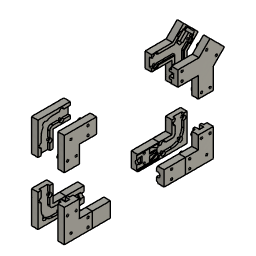
Gabellichtschranke Vorlage v11 (Autodesk Fusion 360 design; units mm, degrees)
Autodesk Fusion 360 part; units mm, degrees
note: some values were not read from the file. Chosen so that the rebuilt part matches the saved one: which bodies a step acts on; which face or edge a step refers to; which pieces of a blend or face edit are solid. Set by a fixed rule: which sketch regions a step uses.
(part 1 of 2)
sketch "Skizze1" plane through (0, 0, 0) normal (1, 0, 0) x (0, 1, 0)
  line L0 (0, 0) -> (80, 0)
  line L1 (80, 0) -> (80, -12)
  line L2 (80, -12) -> (0, -12)
  line L3 (0, -12) -> (0, 0)
  line L4 (0, -12) -> (80, -12)
  line L5 (80, -12) -> (80, -8)
  line L6 (80, -8) -> (0, -8)
  line L7 (0, -8) -> (0, -12)
  line L8 (0, 0) -> (80, 0)
  line L9 (80, 0) -> (80, -4)
  line L10 (0, -4) -> (0, 0)
  line L11 (0, -4) -> (80, -4)
  dimension "d1" = 80
  dimension "d2" = 12
  dimension "d3" = 4
  dimension "d4" = 4
  constraint horizontal L0
  constraint vertical L1
  constraint horizontal L2
  constraint vertical L3
  constraint coincident L0.start L3.end
  constraint horizontal L4
  constraint vertical L5
  constraint horizontal L6
  constraint vertical L7
  constraint coincident L1 L5.end
  constraint horizontal L8
  constraint vertical L9
  constraint vertical L10
  constraint coincident L1 L9.end
  constraint perpendicular L9 L11
  measures "d1" distance of L0.start L0.end
  measures "d2" distance of L0.start L2.end
  measures "d3" distance of L2.end L6.end
  measures "d4" distance of L0.start L10.start
extrude "Extrusion2" add sketch "Skizze1" along normal blind 6 makes body 1
sketch "Skizze2" plane through (0, 0, 0) normal (0, -1, 0) x (1, 0, 0)
  line L0 (0, 0) -> (0, -12)
  line L1 (0, -12) -> (6, -12)
  line L2 (6, -12) -> (6, 0)
  line L3 (6, 0) -> (0, 0)
  circle A0 centre (0, -6) radius 2
  circle A1 centre (0, -6) radius 2.5
  circle A2 centre (0, -6) radius 3
  dimension "d16" = 4
  dimension "d17" = 5
  dimension "d18" = 6
  constraint midpoint L0 A0.centre
  constraint concentric A0 A1
  constraint concentric A0 A2
  measures "d16" diameter of A0
  measures "d17" diameter of A1
  measures "d18" diameter of A2
extrude "Extrusion3" cut sketch "Skizze2" against normal blind 3 contours L0 A0 picked at (0.5038, -5.5634) bodies 1
extrude "Extrusion4" cut sketch "Skizze2" against normal blind 6 from surface at -3 contours L0 A1 A2 | L0 A0 A1 | L0 A0 picked at (0.9319, -8.6687) picked at (0.1186, -3.6751) picked at (0.5038, -5.5634) bodies 1
extrude "Extrusion5" cut sketch "Skizze2" against normal blind 0.8 from surface at -9 contours L0 A0 A1 | L0 A0 picked at (0.1186, -3.6751) picked at (0.5038, -5.5634) bodies 1
extrude "Extrusion6" cut sketch "Skizze2" against normal blind 7 from surface at -9.8 contours L0 A1 A2 | L0 A0 A1 | L0 A0 picked at (0.9319, -8.6687) picked at (0.1186, -3.6751) picked at (0.5038, -5.5634) bodies 1
sketch "Skizze3" plane through (0, 0, 0) normal (-1, 0, 0) x (0, -1, 0)
  line L0 (-9.8, -8.5) -> (-9.8, -9)
  line L1 (-9.8, -9) -> (-16.8, -9)
  line L2 (-16.8, -9) -> (-16.8, -3)
  line L3 (-16.8, -3) -> (-9.8, -3)
  line L4 (-9.8, -3) -> (-9.8, -3.5)
  line L5 (-9.8, -3.5) -> (-9, -3.5)
  line L6 (-9, -3.5) -> (-9, -3)
  line L7 (-9, -3) -> (-3, -3)
  line L8 (-3, -3) -> (-3, -4)
  line L9 (-3, -4) -> (0, -4)
  line L10 (0, -4) -> (0, 0)
  line L11 (0, 0) -> (-80, 0)
  line L12 (-80, 0) -> (-80, -12)
  line L13 (-80, -12) -> (0, -12)
  line L14 (0, -12) -> (0, -8)
  line L15 (0, -8) -> (-3, -8)
  line L16 (-3, -8) -> (-3, -9)
  line L17 (-3, -9) -> (-9, -9)
  line L18 (-9, -9) -> (-9, -8.5)
  line L19 (-9, -8.5) -> (-9.8, -8.5)
  line L20 (-16.8, -6) -> (-19.8, -6)
  line L21 (-19.8, -6) -> (-19.8, -8)
  line L22 (-19.8, -6) -> (-19.8, -4)
  line L23 (-19.8, -4) -> (-80, -4)
  line L24 (-19.8, -8) -> (-80, -8)
  line L25 (-19.8, -4) -> (-19.8, -2)
  line L26 (-19.8, -8) -> (-19.8, -10)
  line L27 (-19.8, -2) -> (-80, -2)
  line L28 (-19.8, -10) -> (-80, -10)
  line L29 (-19.8, -2) -> (-22.8, -2)
  circle A0 centre (-22.8, -2) radius 2
  line L30 (-22.8, -2) -> (-52.8, -2)
  circle A1 centre (-52.8, -2) radius 2
  line L31 (-19.8, -10) -> (-22.8, -10)
  line L32 (-22.8, -10) -> (-52.8, -10)
  circle A2 centre (-52.8, -10) radius 2
  circle A3 centre (-22.8, -10) radius 2
  circle A4 centre (-52.8, -2) radius 1
  circle A5 centre (-22.8, -2) radius 1
  circle A6 centre (-52.8, -10) radius 1
  circle A7 centre (-22.8, -10) radius 1
  circle A8 centre (-22.8, -2) radius 2.75
  circle A9 centre (-52.8, -2) radius 2.75
  circle A10 centre (-52.8, -10) radius 2.75
  circle A11 centre (-22.8, -10) radius 2.75
  dimension "d30" = 3
  dimension "d31" = 2
  dimension "d32" = 2
  dimension "d33" = 2
  dimension "d34" = 2
  dimension "d41" = 3
  dimension "d42" = 4
  dimension "d43" = 30
  dimension "d44" = 4
  dimension "d45" = 3
  dimension "d46" = 30
  dimension "d47" = 4
  dimension "d48" = 4
  dimension "d49" = 2
  dimension "d50" = 2
  dimension "d51" = 2
  dimension "d52" = 2
  dimension "d62" = 5.5
  dimension "d63" = 5.5
  dimension "d64" = 5.5
  dimension "d65" = 5.5
  constraint midpoint L2 L20.start
  constraint perpendicular L2 L20
  constraint perpendicular L1 L21
  constraint perpendicular L20 L22
  constraint coincident L12 L23.end
  constraint perpendicular L12 L23
  constraint coincident L12 L24.end
  constraint perpendicular L12 L24
  constraint perpendicular L23 L25
  constraint perpendicular L24 L26
  constraint coincident L12 L27.end
  constraint perpendicular L12 L27
  constraint coincident L12 L28.end
  constraint perpendicular L12 L28
  constraint perpendicular L25 L29
  constraint coincident L29.end A0.centre
  constraint parallel L27 L30
  constraint coincident L30.end A1.centre
  constraint perpendicular L26 L31
  constraint parallel L28 L32
  constraint coincident L32.end A2.centre
  constraint coincident L31.end L32.start
  constraint concentric A1 A4
  constraint concentric A0 A5
  constraint concentric A2 A6
  constraint concentric A3 A7
  constraint concentric A0 A8
  constraint concentric A4 A9
  constraint concentric A6 A10
  constraint concentric A3 A11
  measures "d30" distance of L20.start L20.end
  measures "d31" distance of L20.end L21.end
  measures "d32" distance of L20.end L22.end
  measures "d33" distance of L22.end L25.end
  measures "d34" distance of L21.end L26.end
  measures "d41" distance of L25.end L29.end
  measures "d42" diameter of A0
  measures "d43" distance of L29.end L30.end
  measures "d44" diameter of A1
  measures "d45" distance of L26.end L31.end
  measures "d46" distance of L31.end L32.end
  measures "d47" diameter of A2
  measures "d48" diameter of A3
  measures "d49" diameter of A4
  measures "d50" diameter of A5
  measures "d51" diameter of A6
  measures "d52" diameter of A7
  measures "d62" diameter of A8
  measures "d63" diameter of A9
  measures "d64" diameter of A10
  measures "d65" diameter of A11
extrude "Extrusion7" add sketch "Skizze3" along normal blind 2 contours L24 L26 L28 L31 A11 | L23 L25 L27 L29 A8 | L24 L28 L31 A3 A11 | L23 L27 L29 A0 A8 | L24 L28 L32 A3 A11 | L28 L31 L32 A3 A7 | L24 L28 L32 A10 A11 | L23 L27 A0 L30 A8 | L27 L29 A0 L30 A5 | L23 L27 L30 A8 A9 | L24 L28 L32 A2 A10 | L23 L27 L30 A1 A9 | L28 L31 L32 A7 | L24 L28 A2 A10 | L28 L32 A2 A6 | L12 L24 L28 A10 | L27 L29 L30 A5 | L23 L27 A1 A9 | L27 L30 A1 A4 | L12 L23 L27 A9 | L28 L32 A6 | L27 L30 A4 picked at (-22.9198, -8.3411) picked at (-22.9198, -3.6589) picked at (-23.3198, -9.5855) picked at (-52.9198, -8.3411) picked at (-22.1371, -2.0497) picked at (-52.9198, -3.6589) picked at (-52.3478, -9.5127) picked at (-52.1371, -2.0497) bodies 1
extrude "Extrusion8" cut sketch "Skizze3" against normal blind 2 contours L12 L21 L22 L23 L24 A8 A9 A10 A11 | L24 A11 | L23 A8 | L24 A10 | L23 A9 bodies 1
extrude "Extrusion9" cut 1 faces at (0.6667, 19.8, -6.6667) along direction (0, -1, 0) blind 6 on bodies 1 bodies 1
extrude "Extrusion10" add sketch "Skizze3" along normal blind 2 contours L28 L31 L32 A3 A7 | L27 L29 A0 L30 A5 | L28 L31 L32 A7 | L27 L29 L30 A5 | L28 L32 A2 A6 | L27 L30 A1 A4 | L28 L32 A6 | L27 L30 A4 picked at (-22.9198, -11.6589) picked at (-22.9198, -0.3411) picked at (-23.4629, -10.0497) picked at (-23.4629, -1.9503) picked at (-52.9198, -11.6589) picked at (-52.9198, -0.3411) picked at (-53.4629, -10.0497) picked at (-53.4629, -1.9503) bodies 1
extrude "Extrusion11" cut 1 faces at (4.6667, 80, -5.3333) along direction (0, -1, 0) blind 22 on bodies 1 bodies 1
copy_body "Körper kopieren/einfügen1" bodies 1 makes body 2
move_body "Verschieben1" bodies 2 to x (1, 0, 0) y (0, 1, 0) z (0, 0, 1) at (-33, 0, 0)
extrude "Extrusion12" cut 2 faces at (-35, 34.2, -8.6667) (-35, 42.8667, -3.3333) along direction (1, 0, 0) blind 4 on bodies 2 bodies 2
extrude "Extrusion13" cut sketch "Skizze3" along normal blind 100 from surface at -10 contours L28 L31 L32 A7 | L28 L31 L32 A7 | L27 L29 L30 A5 | L27 L29 L30 A5 | L28 L32 A6 | L28 L32 A6 | L27 L30 A4 | L27 L30 A4 bodies 1 2
extrude "Extrusion14" add 2 faces at (4, 26.9333, 0) (-30.3333, 7.6, 0) along direction (0, 0, 1) blind 1 on bodies 1 2 bodies 1 2
extrude "Extrusion15" add 2 faces at (4, 26.9333, -12) (-30.3333, 7.6, -12) along direction (0, 0, -1) blind 1 on bodies 1 2 bodies 1 2
extrude "Extrusion16" cut sketch "Skizze3" against normal blind 3 from surface at -3 contours L24 L28 L31 A3 A11 | L24 A11 | L23 A8 | L23 L27 L29 A0 A8 | L24 L28 L32 A3 A11 | L28 L31 L32 A3 A7 | L13 L28 L31 A3 A11 | L23 L27 A0 L30 A8 | L27 L29 A0 L30 A5 | L11 L27 L29 A0 A8 | L13 A11 | L28 L31 L32 A3 A7 | L13 L28 L32 A3 A11 | L24 L28 L32 A2 A10 | L24 A10 | L27 L29 A0 L30 A5 | L11 L27 A0 L30 A8 | L23 A9 | L23 L27 L30 A1 A9 | L11 A8 | L28 L31 L32 A7 | L28 L31 L32 A7 | L24 L28 A2 A10 | L28 L32 A2 A6 | L13 L28 L32 A2 A10 | L27 L29 L30 A5 | L27 L29 L30 A5 | L23 L27 A1 A9 | L27 L30 A1 A4 | L11 L27 L30 A1 A9 | L13 A10 | L28 L32 A2 A6 | L13 L28 A2 A10 | L27 L30 A1 A4 | L11 L27 A1 A9 | L11 A9 | L28 L32 A6 | L28 L32 A6 | L27 L30 A4 | L27 L30 A4 bodies 1
move_body "Verschieben2" bodies 2 to x (-1, 0, 0) y (0, 1, 0) z (0, 0, -1) at (-66, 0, -26)
move_body "Verschieben3" bodies 2 to x (1, 0, 0) y (0, 1, 0) z (0, 0, 1) at (33, 0, 14)
move_body "Verschieben4" bodies 2 to x (1, 0, 0) y (0, 1, 0) z (0, 0, 1) at (-12, 0, 0)
copy_body "Körper kopieren/einfügen2" bodies 1 makes body 3
move_body "Verschieben5" bodies 3 to x (1, 0, 0) y (0, 1, 0) z (0, 0, 1) at (-52, 0, 0)
extrude "Extrusion17" cut 1 faces at (-47.3352, 0, -6.0498) along direction (0, 1, 0) blind 18 on bodies 3 bodies 3
extrude "Extrusion18" add 1 faces at (-47.3333, 18, -5.3333) along direction (0, -1, 0) blind 18 on bodies 3 bodies 3
sketch "Skizze4" plane through (-52, 0, 0) normal (-1, 0, 0) x (0, -1, 0)
  line L0 (0, -8) -> (-19.8, -8)
  line L1 (-19.8, -8) -> (-19.8, -10)
  line L2 (-19.8, -10) -> (-20.8, -10)
  arc A0 (-24.8, -10) -> (-20.8, -10) centre (-22.8, -10) ccw
  line L3 (-24.8, -10) -> (-50.8, -10)
  arc A1 (-54.8, -10) -> (-50.8, -10) centre (-52.8, -10) ccw
  line L4 (-54.8, -10) -> (-58, -10)
  line L5 (-58, -10) -> (-58, -13)
  line L6 (-58, -13) -> (0, -13)
  line L7 (0, -13) -> (0, -8)
  line L8 (-16, -8) -> (-19.8, -8)
  line L9 (-19.8, -8) -> (-19.8, -4)
  line L10 (-19.8, -4) -> (-16, -4)
  line L11 (0, -4) -> (0, -8)
  line L12 (0, -6) -> (-19.8, -6) construction
  line L13 (0, -6) -> (-2, -6)
  line L14 (-2, -6) -> (-2, -8.75)
  line L15 (-2, -6) -> (-2, -3.25)
  line L16 (-2, -3.25) -> (-5, -3.25)
  line L17 (-5, -3.25) -> (-5, -8.75)
  line L18 (-5, -8.75) -> (-2, -8.75)
  line L19 (-2, -8.75) -> (-2, -3.25)
  line L20 (-5, -6) -> (-5, -7.25)
  line L21 (-5, -7.25) -> (-10, -7.25)
  line L22 (-10, -7.25) -> (-10, -4.75)
  line L23 (-10, -4.75) -> (-5, -4.75)
  line L24 (-5, -4.75) -> (-5, -7.25)
  line L25 (-5, -7.25) -> (-5, -8.25)
  line L26 (-5, -4.75) -> (-5, -3.75)
  line L27 (-5, -8.25) -> (-8, -8.25)
  line L28 (-5, -3.75) -> (-8, -3.75)
  line L29 (-9, -9.25) -> (-9, -10.25)
  line L30 (-10, -7.25) -> (-10, -9.25)
  line L31 (-11, -10.25) -> (-13, -10.25)
  line L32 (-14, -9.25) -> (-14, -7.25)
  line L33 (-10, -4.75) -> (-10, -2.75)
  line L34 (-9, -2.75) -> (-9, -1.75)
  line L35 (-11, -1.75) -> (-13, -1.75)
  line L36 (-14, -2.75) -> (-14, -7.25)
  line L37 (-10, -0.75) -> (-14, -0.75)
  line L38 (-15, -1.75) -> (-15, -3)
  line L39 (-10, -11.25) -> (-14, -11.25)
  line L40 (-15, -10.25) -> (-15, -9)
  line L41 (-14, -6) -> (-14, -6.75)
  line L42 (-14, -6) -> (-14, -5.25)
  line L43 (-16.8, -4) -> (-16.8, -8)
  line L44 (-14, -6.75) -> (-16.8, -6.75)
  line L45 (-14, -5.25) -> (-16.8, -5.25)
  arc A2 (-8, -8.25) -> (-9, -9.25) centre (-8, -9.25) ccw
  arc A3 (-11, -10.25) -> (-10, -9.25) centre (-11, -9.25) ccw
  arc A4 (-14, -9.25) -> (-13, -10.25) centre (-13, -9.25) ccw
  arc A5 (-15, -9) -> (-16, -8) centre (-16, -9) ccw
  arc A6 (-9, -2.75) -> (-8, -3.75) centre (-8, -2.75) ccw
  arc A7 (-10, -2.75) -> (-11, -1.75) centre (-11, -2.75) ccw
  arc A8 (-13, -1.75) -> (-14, -2.75) centre (-13, -2.75) ccw
  arc A9 (-16, -4) -> (-15, -3) centre (-16, -3) ccw
  arc A10 (-9, -1.75) -> (-10, -0.75) centre (-10, -1.75) ccw
  arc A11 (-14, -0.75) -> (-15, -1.75) centre (-14, -1.75) ccw
  arc A12 (-15, -10.25) -> (-14, -11.25) centre (-14, -10.25) ccw
  arc A13 (-10, -11.25) -> (-9, -10.25) centre (-10, -10.25) ccw
  point P0 (-19.8, -4)
  point P1 (-9, -8.25)
  point P2 (-9, -3.75)
  point P3 (-9, -11.25)
  point P4 (-10, -10.25)
  point P5 (-14, -10.25)
  point P6 (-10, -1.75)
  point P7 (-9, -0.75)
  point P8 (-14, -1.75)
  point P9 (-15, -0.75)
  dimension "d79" = 2
  dimension "d80" = 2.75
  dimension "d81" = 2.75
  dimension "d82" = 3
  dimension "d83" = 5.5
  dimension "d84" = 1.25
  dimension "d85" = 5
  dimension "d86" = 2.5
  dimension "d87" = 1
  dimension "d88" = 1
  dimension "d89" = 4
  dimension "d90" = 4
  dimension "d92" = 3
  dimension "d93" = 4
  dimension "d94" = 3
  dimension "d95" = 3
  dimension "d96" = 4
  dimension "d97" = 6
  dimension "d107" = 0.75
  dimension "d108" = 0.75
  dimension "d113" = 1
  dimension "d118" = 1
  constraint horizontal L8
  constraint vertical L9
  constraint horizontal L10
  constraint vertical L11
  constraint coincident P0 L9.end
  constraint coincident L0.start L7.end
  constraint midpoint L11 L12.start
  constraint midpoint L9 L12.end
  constraint perpendicular L11 L13
  constraint perpendicular L13 L14
  constraint perpendicular L12 L15
  constraint horizontal L16
  constraint vertical L17
  constraint horizontal L18
  constraint vertical L19
  constraint midpoint L17 L20.start
  constraint perpendicular L12 L20
  constraint horizontal L21
  constraint vertical L22
  constraint horizontal L23
  constraint vertical L24
  constraint perpendicular L21 L25
  constraint perpendicular L10 L26
  constraint perpendicular L25 L27
  constraint perpendicular L17 L28
  constraint perpendicular L8 L29
  constraint perpendicular L8 L30
  constraint perpendicular L30 L31
  constraint perpendicular L21 L32
  constraint perpendicular L10 L33
  constraint perpendicular L28 L34
  constraint perpendicular L33 L35
  constraint perpendicular L34 L37
  constraint vertical L38
  constraint perpendicular L29 L39
  constraint coincident L36 L41.start
  constraint coincident L12 L41.start
  constraint perpendicular L12 L41
  constraint perpendicular L12 L42
  constraint coincident L43 L44.end
  constraint perpendicular L36 L44
  constraint horizontal L45
  constraint coincident L43 L45.end
  constraint coincident P1 L29
  constraint coincident P1 L27
  constraint tangent L29 A2
  constraint tangent L27 A2
  constraint coincident P4 L31
  constraint coincident P4 L30
  constraint tangent L31 A3
  constraint tangent L30 A3
  constraint equal A2 A3
  constraint coincident P5 L31
  constraint coincident P5 L32
  constraint tangent L31 A4
  constraint tangent L32 A4
  constraint equal A2 A4
  constraint coincident L0.start L8
  constraint tangent L40 A5
  constraint tangent L8 A5
  constraint equal A2 A5
  constraint coincident P2 L28
  constraint coincident P2 L34
  constraint tangent L28 A6
  constraint tangent L34 A6
  constraint equal A2 A6
  constraint coincident P6 L33
  constraint coincident P6 L35
  constraint tangent L33 A7
  constraint tangent L35 A7
  constraint equal A2 A7
  constraint coincident P8 L35
  constraint coincident P8 L36
  constraint tangent L35 A8
  constraint tangent L36 A8
  constraint equal A2 A8
  constraint coincident L11.start L10
  constraint tangent L10 A9
  constraint tangent L38 A9
  constraint equal A2 A9
  constraint coincident P7 L34
  constraint coincident P7 L37
  constraint tangent L34 A10
  constraint tangent L37 A10
  constraint coincident P9 L37
  constraint coincident P9 L38
  constraint tangent L37 A11
  constraint tangent L38 A11
  constraint equal A10 A11
  constraint tangent L40 A12
  constraint tangent L39 A12
  constraint equal A10 A12
  constraint coincident P3 L39
  constraint coincident P3 L29
  constraint tangent L39 A13
  constraint tangent L29 A13
  constraint equal A10 A13
  measures "d79" distance of L12.start L13.end
  measures "d80" distance of L13.end L14.end
  measures "d81" distance of L13.end L15.end
  measures "d82" distance of L15.end L16.end
  measures "d83" distance of L15.end L14.end
  measures "d84" distance of L20.start L20.end
  measures "d85" distance of L20.end L21.end
  measures "d86" distance of L20.end L23.end
  measures "d87" distance of L20.end L25.end
  measures "d88" distance of L23.end L26.end
  measures "d89" distance of L25.end P1
  measures "d90" distance of L26.end P2
  measures "d92" distance of L21.end P4
  measures "d93" distance of P4 P5
  measures "d94" distance of L22.end P6
  measures "d95" distance of P2 P7
  measures "d96" distance of P6 P8
  measures "d97" distance of P7 P9
  measures "d107" distance of L41.start L41.end
  measures "d108" distance of L41.start L42.end
  measures "d113" radius of A2
  measures "d118" radius of A10
extrude "Extrusion19" add sketch "Skizze4" against normal blind 2 contours L0 L8 L9 L10 L43 bodies 3
extrude "Extrusion21" cut sketch "Skizze4" against normal blind 1 contours L0 L17 L25 L27 L29 L30 L31 L32 L39 L40 A2 A3 A4 A5 A12 A13 | L0 L17 L21 L25 L30 | L10 L17 L23 L26 L28 L33 L34 L35 L36 L37 L38 L43 L45 A6 A7 A8 A9 A10 A11 bodies 3
extrude "Extrusion22" cut sketch "Skizze4" against normal blind 2.5 contours L0 L14 L15 L16 L17 L19 L20 L24 L25 L26 | L0 L14 L17 L18 L19 L25 bodies 3
extrude "Extrusion23" cut sketch "Skizze4" against normal blind 2 contours L0 L8 L9 L10 L43 bodies 3
extrude "Extrusion25" add sketch "Skizze4" against normal blind 2 contours L36 L41 L42 L43 L44 L45 bodies 3
extrude "Extrusion26" add sketch "Skizze4" against normal blind 2 contours L0 L22 L30 L32 L33 L35 L36 L41 L42 A7 A8 | L17 L20 L21 L22 L23 L24 bodies 3
extrude "Extrusion27" add 2 faces at (-50, 8.3333, -7.5) (-50, 8.3333, -4.25) along direction (-1, 0, 0) blind 1 on bodies 3 bodies 3
extrude "Extrusion28" add 1 faces at (-50, 1.3333, -5.3333) along direction (-1, 0, 0) blind 2 on bodies 3 bodies 3
sketch "Skizze5" plane through (0, 0, 0) normal (0, -1, 0) x (1, 0, 0)
  line L0 (-52, 1) -> (-52, -13)
  line L1 (-52, -13) -> (-46, -13)
  line L2 (-46, -13) -> (-46, 1)
  line L3 (-46, 1) -> (-52, 1)
  circle A0 centre (-52, -6) radius 2.25
  dimension "d121" = 4.5
  constraint midpoint L0 A0.centre
  measures "d121" diameter of A0
extrude "Extrusion29" cut sketch "Skizze5" against normal blind 2 contours L0 A0 picked at (-50.8857, -5.4332) bodies 3
copy_body "Körper kopieren/einfügen3" bodies 3 makes body 4
move_body "Verschieben6" bodies 4 to x (-1, 0, 0) y (0, 1, 0) z (0, 0, -1) at (-149, 0, -26)
move_body "Verschieben7" bodies 4 to x (1, 0, 0) y (0, 1, 0) z (0, 0, 1) at (45, 0, 14)
move_body "Verschieben8" bodies 4 to x (1, 0, 0) y (0, 1, 0) z (0, 0, 1) at (-53, 0, 0)
extrude "Extrusion30" cut 2 faces at (-103, 56.9333, -9.3333) (-103, 56.9333, -2.6667) along direction (-1, 0, 0) blind 4 on bodies 4 bodies 4
extrude "Extrusion31" add 4 faces at (-108, 50.6436, -10.1366) (-108, 20.6473, -10.1863) (-108, 20.6473, -1.8137) (-108, 50.6473, -2.1863) along direction (-1, 0, 0) blind 3 on bodies 4 bodies 4
move_body "Verschieben9" bodies 1 to x (1, 0, 0) y (0, 1, 0) z (0, 0, 1) at (-12, 0, 0)
sketch "Skizze6" plane through (0, 0, 0) normal (0, -1, 0) x (1, 0, 0)
  arc A0 (-12, -8) -> (-12, -4) centre (-12, -6) ccw
  line L0 (-12, -8) -> (-12, -13)
  line L1 (-12, -13) -> (-6, -13)
  line L2 (-6, -13) -> (-6, 1)
  line L3 (-6, 1) -> (-12, 1)
  line L4 (-12, 1) -> (-12, -4)
  circle A1 centre (-12, -6) radius 4
  dimension "d128" = 8
  constraint concentric A0 A1
  measures "d128" diameter of A1
extrude "Extrusion32" cut sketch "Skizze6" against normal blind 7 from surface at -9.8 contours A0 L0 L4 A1 | A0 L0 L4 A1 bodies 1 2
move_body "Verschieben10" bodies 1 to x (1, 0, 0) y (0, 1, 0) z (0, 0, 1) at (22, 0, 0)
chamfer "Fase1" distance 0.5 angle 45 12 edges at (-12, 22.8, 0) (-12, 52.8, 0) (-12, 52.8, -12) (-12, 22.8, -12) (-12, 37.8, -2) (-12, 56.4, -2) (-12, 56.4, -10) (-12, 37.8, -10) (-12, 20.3, -10) (-12, 19.8, -9) (-12, 19.8, -3) (-12, 20.3, -2) on bodies 2
chamfer "Fase2" distance 0.5 angle 45 16 edges at (8, 52.8, -12) (8, 22.8, -12) (8, 37.8, -10) (8, 56.4, -10) (8, 20.3, -10) (8, 22.8, 0) (8, 37.8, -2) (8, 56.4, -2) (8, 19.8, -9) (8, 58, -9) (8, 58, -3) (8, 52.8, 0) (10, 52.8, 0) (10, 22.8, 0) (8, 20.3, -2) (8, 19.8, -3) on bodies 1
extrude "Extrusion33" add 4 faces at (13, 54.2878, -8.4331) (13, 53.1467, -4.1328) (13, 20.6473, -9.8137) (13, 20.6473, -1.8137) along direction (1, 0, 0) blind 3 on bodies 1 bodies 1
chamfer "Fase3" distance 2 angle 45 4 edges at (16, 53.7323, -10.3616) (16, 53.7323, -2.3616) (16, 23.7323, -2.3616) (16, 23.7323, -10.3616) on bodies 1
sketch "Skizze7" plane through (-105, 0, 0) normal (1, 0, 0) x (0, 1, 0)
  line L0 (10, -2.75) -> (10, -4.75)
  line L1 (10, -4.75) -> (5, -4.75)
  line L2 (5, -4.75) -> (5, -7.25)
  line L3 (5, -7.25) -> (10, -7.25)
  line L4 (10, -7.25) -> (10, -9.25)
  arc A0 (10, -9.25) -> (11, -10.25) centre (11, -9.25) ccw
  line L5 (11, -10.25) -> (13, -10.25)
  arc A1 (13, -10.25) -> (14, -9.25) centre (13, -9.25) ccw
  line L6 (14, -9.25) -> (14, -6.75)
  line L7 (14, -6.75) -> (16.8, -6.75)
  line L8 (16.8, -6.75) -> (16.8, -5.25)
  line L9 (16.8, -5.25) -> (14, -5.25)
  line L10 (14, -5.25) -> (14, -2.75)
  arc A2 (14, -2.75) -> (13, -1.75) centre (13, -2.75) ccw
  line L11 (13, -1.75) -> (11, -1.75)
  arc A3 (11, -1.75) -> (10, -2.75) centre (11, -2.75) ccw
  line L12 (10, -4.75) -> (14, -4.75)
  line L13 (14, -4.75) -> (14, -1.75)
  line L14 (14, -1.75) -> (10, -1.75)
  line L15 (10, -1.75) -> (10, -4.75)
  line L16 (12, -1.75) -> (12, -3.75)
  circle A4 centre (12, -3.75) radius 2
  line L17 (12, -10.25) -> (12, -8.25)
  circle A5 centre (12, -8.25) radius 2
  dimension "d137" = 2
  dimension "d140" = 2
  constraint horizontal L12
  constraint vertical L13
  constraint horizontal L14
  constraint vertical L15
  constraint coincident L0.end L1.start
  constraint midpoint L11 L16.start
  constraint perpendicular L14 L16
  constraint coincident L16.end A4.centre
  constraint coincident L16.start A4
  constraint tangent L14 A4
  constraint midpoint L5 L17.start
  constraint perpendicular L5 L17
  constraint coincident L17.end A5.centre
  constraint coincident L17.start A5
  measures "d137" distance of L16.start L16.end
  measures "d140" distance of L17.start L17.end
extrude "Extrusion34" cut sketch "Skizze7" against normal blind 1 contours L0 L11 A3 L14 L15 A4 | L10 A2 L11 L13 L14 A4 bodies 4
extrude "Extrusion36" cut sketch "Skizze7" against normal blind 1 contours L4 A0 L5 A5 | L5 A1 L6 A5 bodies 4
sketch "Skizze8" plane through (-52, 0, 0) normal (-1, 0, 0) x (0, -1, 0)
  line L0 (-10, -9.25) -> (-10, -7.25)
  line L1 (-10, -7.25) -> (-5, -7.25)
  line L2 (-5, -7.25) -> (-5, -4.75)
  line L3 (-5, -4.75) -> (-10, -4.75)
  line L4 (-10, -4.75) -> (-10, -2.75)
  arc A0 (-10, -2.75) -> (-11, -1.75) centre (-11, -2.75) ccw
  line L5 (-11, -1.75) -> (-13, -1.75)
  arc A1 (-13, -1.75) -> (-14, -2.75) centre (-13, -2.75) ccw
  line L6 (-14, -2.75) -> (-14, -5.25)
  line L7 (-14, -5.25) -> (-16.8, -5.25)
  line L8 (-16.8, -5.25) -> (-16.8, -6.75)
  line L9 (-16.8, -6.75) -> (-14, -6.75)
  line L10 (-14, -6.75) -> (-14, -9.25)
  arc A2 (-14, -9.25) -> (-13, -10.25) centre (-13, -9.25) ccw
  line L11 (-13, -10.25) -> (-11, -10.25)
  arc A3 (-11, -10.25) -> (-10, -9.25) centre (-11, -9.25) ccw
  line L12 (-12, -10.25) -> (-12, -8.25)
  line L13 (-12, -1.75) -> (-12, -3.75)
  circle A4 centre (-12, -3.75) radius 2
  circle A5 centre (-12, -8.25) radius 2
  line L14 (-12, -1.75) -> (-12, -10.25)
  line L15 (-14, -5.25) -> (-12, -5.25)
  line L16 (-14, -6.75) -> (-12, -6.75)
  dimension "d145" = 2
  dimension "d146" = 2
  constraint midpoint L11 L12.start
  constraint perpendicular L11 L12
  constraint midpoint L5 L13.start
  constraint perpendicular L5 L13
  constraint coincident L13.end A4.centre
  constraint coincident L13.start A4
  constraint coincident L12.end A5.centre
  constraint coincident L12.start A5
  constraint coincident L6.end L7.start
  constraint coincident L14 L15.end
  constraint perpendicular L14 L15
  constraint coincident L9.end L10.start
  constraint coincident L14 L16.end
  constraint perpendicular L14 L16
  measures "d145" distance of L12.start L12.end
  measures "d146" distance of L13.start L13.end
extrude "Extrusion37" cut sketch "Skizze8" against normal blind 1 contours L0 L11 A3 A5 | L10 A2 L11 A5 | L4 A0 L5 A4 | L5 A1 L6 A4 bodies 3
sketch "Skizze9" plane through (-52, 0, 0) normal (-1, 0, 0) x (0, -1, 0)
  line L0 (0, -8.25) -> (-2, -8.25)
  line L1 (-2, -8.25) -> (-2, -8.75)
  line L2 (-2, -8.75) -> (-5, -8.75)
  line L3 (-5, -8.75) -> (-5, -8.25)
  line L4 (-5, -8.25) -> (-8, -8.25)
  arc A0 (-8, -8.25) -> (-9, -9.25) centre (-8, -9.25) ccw
  line L5 (-9, -9.25) -> (-9, -10.25)
  arc A1 (-10, -11.25) -> (-9, -10.25) centre (-10, -10.25) ccw
  line L6 (-10, -11.25) -> (-14, -11.25)
  arc A2 (-15, -10.25) -> (-14, -11.25) centre (-14, -10.25) ccw
  line L7 (-15, -10.25) -> (-15, -9)
  arc A3 (-15, -9) -> (-16, -8) centre (-16, -9) ccw
  line L8 (-16, -8) -> (-19.8, -8)
  line L9 (-19.8, -8) -> (-19.8, -10)
  line L10 (-19.8, -10) -> (-20.8, -10)
  arc A4 (-24.8, -10) -> (-20.8, -10) centre (-22.8, -10) ccw
  line L11 (-24.8, -10) -> (-50.8, -10)
  arc A5 (-54.8, -10) -> (-50.8, -10) centre (-52.8, -10) ccw
  line L12 (-54.8, -10) -> (-58, -10)
  line L13 (-58, -10) -> (-58, -13)
  line L14 (-58, -13) -> (0, -13)
  line L15 (0, -13) -> (0, -8.25)
  line L16 (-19.8, -8) -> (0, -8)
  line L17 (0, -8) -> (0, -12)
  line L18 (0, -12) -> (-17.8, -12)
  line L19 (-19.8, -10) -> (-19.8, -8)
  circle A6 centre (-7, -10) radius 1
  line L20 (-19.8, -10) -> (-17.8, -10)
  arc A7 (-19.8, -10) -> (-17.8, -12) centre (-17.8, -10) ccw
  dimension "d152" = 2
  constraint horizontal L16
  constraint vertical L17
  constraint horizontal L18
  constraint vertical L19
  constraint coincident L8.end L9.start
  constraint coincident L9.end L10.start
  constraint perpendicular L19 L20
  constraint coincident L20.end A7.centre
  constraint tangent L18 A7
  measures "d152" distance of L9.end L20.end
extrude "Extrusion38" add sketch "Skizze9" along normal blind 1 contours L0 L1 L2 L3 L4 A0 L5 A1 L6 A2 L7 A3 L8 L9 L15 L16 L17 L18 L19 A7 bodies 3
extrude "Extrusion39" cut 1 faces at (-52, 7.2865, -9.7637) along direction (1, 0, 0) blind 6 on bodies 3 bodies 3
extrude "Extrusion40" add sketch "Skizze8" along normal blind 1 contours L0 L1 L2 L3 L4 A4 A5 L14 | L12 A5 L14 | L12 A5 L14 L16 | A5 L14 L16 | L7 L8 L9 A4 A5 L14 L15 L16 | L10 A5 L16 | L13 A4 L14 | A4 L14 L15 | L6 A4 L15 | L13 A4 L14 L15 bodies 3
sketch "Skizze10" plane through (-52, 0, 0) normal (-1, 0, 0) x (0, -1, 0)
  line L0 (-2, -3.75) -> (0, -3.75)
  line L1 (0, -3.75) -> (0, 1)
  line L2 (0, 1) -> (-58, 1)
  line L3 (-58, 1) -> (-58, -2)
  line L4 (-58, -2) -> (-54.8, -2)
  arc A0 (-50.8, -2) -> (-54.8, -2) centre (-52.8, -2) ccw
  line L5 (-50.8, -2) -> (-24.8, -2)
  arc A1 (-20.8, -2) -> (-24.8, -2) centre (-22.8, -2) ccw
  line L6 (-20.8, -2) -> (-19.8, -2)
  line L7 (-19.8, -2) -> (-19.8, -4)
  line L8 (-19.8, -4) -> (-16, -4)
  arc A2 (-16, -4) -> (-15, -3) centre (-16, -3) ccw
  line L9 (-15, -3) -> (-15, -1.75)
  arc A3 (-14, -0.75) -> (-15, -1.75) centre (-14, -1.75) ccw
  line L10 (-14, -0.75) -> (-10, -0.75)
  arc A4 (-9, -1.75) -> (-10, -0.75) centre (-10, -1.75) ccw
  line L11 (-9, -1.75) -> (-9, -2.75)
  arc A5 (-9, -2.75) -> (-8, -3.75) centre (-8, -2.75) ccw
  line L12 (-8, -3.75) -> (-5, -3.75)
  line L13 (-5, -3.75) -> (-5, -3.25)
  line L14 (-5, -3.25) -> (-2, -3.25)
  line L15 (-2, -3.25) -> (-2, -3.75)
  line L16 (-19.8, -4) -> (0, -4)
  line L17 (0, -4) -> (0, 0)
  line L18 (0, 0) -> (-17.8, 0)
  line L19 (-19.8, -2) -> (-19.8, -4)
  circle A6 centre (-7, -2) radius 1
  arc A7 (-17.8, 0) -> (-19.8, -2) centre (-17.8, -2) ccw
  line L20 (-19.8, -4) -> (-14, -0.75)
  line L21 (-14, -4) -> (-14, -0.75)
  point P0 (-14, -4)
  dimension "d161" = 2
  constraint horizontal L16
  constraint vertical L17
  constraint horizontal L18
  constraint vertical L19
  constraint coincident L7.end L8.start
  constraint tangent L18 A7
  constraint coincident A3.start L10.start
  constraint coincident P0 L21.start
  measures "d161" diameter of A6
extrude "Extrusion41" add sketch "Skizze10" against normal blind 1 contours A3 L20 bodies 3
extrude "Extrusion42" cut sketch "Skizze10" against normal blind 2 contours A2 L9 A3 L16 L20 L21 | L8 A2 L9 A3 L16 L20 bodies 3
extrude "Extrusion43" add 1 faces at (-52, 16.8, -6.25) along direction (0, 1, 0) blind 3 on bodies 3 bodies 3
extrude "Extrusion44" cut 1 faces at (-52, 19.8, -6.25) along direction (0, -1, 0) blind 1.5 on bodies 3 bodies 3
sketch "Skizze11" plane through (-53, 0, 0) normal (-1, 0, 0) x (0, -1, 0)
  line L0 (-18.3, -5.25) -> (-18.3, -6.75)
  line L1 (-18.3, -6.75) -> (-14, -6.75)
  line L2 (-14, -6.75) -> (-14, -8.25)
  arc A0 (-14, -8.25) -> (-10, -8.25) centre (-12, -8.25) ccw
  line L3 (-10, -8.25) -> (-10, -7.25)
  line L4 (-10, -7.25) -> (-5, -7.25)
  line L5 (-5, -7.25) -> (-5, -4.75)
  line L6 (-5, -4.75) -> (-10, -4.75)
  line L7 (-10, -4.75) -> (-10, -3.75)
  arc A1 (-10, -3.75) -> (-14, -3.75) centre (-12, -3.75) ccw
  line L8 (-14, -3.75) -> (-14, -5.25)
  line L9 (-14, -5.25) -> (-18.3, -5.25)
  line L10 (-14, -0.75) -> (-10, -0.75)
  line L11 (-10, -11.25) -> (-14, -11.25)
  line L12 (-12, -0.75) -> (-12, -11.25)
  line L13 (-12, -0.75) -> (-14, -0.75)
  line L14 (-14, -0.75) -> (-14, -11.25)
  line L15 (-12, -11.25) -> (-14, -11.25)
  constraint midpoint L10 L12.start
  constraint midpoint L11 L12.end
  constraint coincident L10.start L13.end
  constraint coincident L11.end L14.end
extrude "Extrusion47" cut sketch "Skizze11" against normal blind 3 contours L2 A0 A1 L8 L12 L14 | A1 L10 L12 L13 L14 | A0 L11 L12 L14 L15 bodies 3
extrude "Extrusion48" add 1 faces at (-52, 14, -5.75) along direction (0, -1, 0) blind 2 on bodies 3 bodies 3
sketch "Skizze12" plane through (-53, 0, 0) normal (-1, 0, 0) x (0, -1, 0)
  circle A0 centre (-7, -10) radius 1
  line L0 (-19.8, -8) -> (-19.8, -10)
  arc A1 (-19.8, -10) -> (-17.8, -12) centre (-17.8, -10) ccw
  line L1 (-17.8, -12) -> (0, -12)
  line L2 (0, -12) -> (0, -8.25)
  line L3 (0, -8.25) -> (-2, -8.25)
  line L4 (-2, -8.25) -> (-2, -8.75)
  line L5 (-2, -8.75) -> (-5, -8.75)
  line L6 (-5, -8.75) -> (-5, -8.25)
  line L7 (-5, -8.25) -> (-8, -8.25)
  arc A2 (-8, -8.25) -> (-9, -9.25) centre (-8, -9.25) ccw
  line L8 (-9, -9.25) -> (-9, -10.25)
  arc A3 (-10, -11.25) -> (-9, -10.25) centre (-10, -10.25) ccw
  line L9 (-10, -11.25) -> (-14, -11.25)
  arc A4 (-15, -10.25) -> (-14, -11.25) centre (-14, -10.25) ccw
  line L10 (-15, -10.25) -> (-15, -9)
  arc A5 (-15, -9) -> (-16, -8) centre (-16, -9) ccw
  line L11 (-16, -8) -> (-19.8, -8)
  line L12 (-14, -11.25) -> (-19.8, -8)
  constraint coincident L9.end A4.end
  constraint coincident L0.start L11.end
extrude "Extrusion49" add sketch "Skizze12" against normal blind 2 contours A4 L12 bodies 3
extrude "Extrusion50" cut sketch "Skizze12" against normal blind 3 contours A4 L10 A5 L11 L12 bodies 3
extrude "Extrusion51" cut 1 faces at (-51, 14.3333, -9.4167) along direction (1, 0, 0) blind 1 on bodies 3 bodies 3
extrude "Extrusion52" add sketch "Skizze10" along normal blind 1 contours L0 L1 L7 A3 L10 A4 L11 A5 L12 L13 L14 L15 L17 L18 L19 A7 L20 | A3 L20 bodies 3
extrude "Extrusion53" cut sketch "Skizze10" against normal blind 6 contours A6 bodies 3
extrude "Extrusion54" cut 2 faces at (-53, 2.6997, -1.6054) (-53, 2.6997, -10.3946) along direction (-1, 0, 0) blind 1 from surface at 52 on bodies 3 bodies 4
extrude "Extrusion55" cut 5 faces at (-105, 6.8671, -2.4582) (-105, 7.2754, -9.9116) (-105, 16.9333, -3.25) (-105, 16.9333, -8.75) (-105, 8.3333, -5.5833) along direction (-1, 0, 0) blind 1 on bodies 4 bodies 4
extrude "Extrusion56" cut 1 faces at (-105.3333, 1.3333, -3.75) along direction (0, 0, -1) blind 5.4 on bodies 4 bodies 4
extrude "Extrusion57" cut 1 faces at (-50, 45.2667, -6.6667) along direction (-1, 0, 0) blind 57 on bodies 3 bodies 4
sketch "Skizze13" plane through (-106, 0, 0) normal (1, 0, 0) x (0, 1, 0)
  line L0 (16.8, -5.25) -> (12, -5.25)
  line L1 (12, -5.25) -> (12, -0.75)
  line L2 (12, -0.75) -> (14, -0.75)
  line L3 (14, -0.75) -> (19.8, -4)
  line L4 (19.8, -4) -> (19.8, -2)
  arc A0 (19.8, -2) -> (17.8, 0) centre (17.8, -2) ccw
  line L5 (17.8, 0) -> (0, 0)
  line L6 (0, 0) -> (0, -3.9844)
  line L7 (0, -3.9844) -> (2, -3.9844)
  line L8 (2, -3.9844) -> (2, -3.25)
  line L9 (2, -3.25) -> (5, -3.25)
  line L10 (5, -3.25) -> (5, -8.75)
  line L11 (5, -8.75) -> (2, -8.75)
  line L12 (2, -8.75) -> (2, -8.0156)
  line L13 (2, -8.0156) -> (0, -8.0156)
  line L14 (0, -8.0156) -> (0, -12)
  line L15 (0, -12) -> (17.8, -12)
  arc A1 (17.8, -12) -> (19.8, -10) centre (17.8, -10) ccw
  line L16 (19.8, -10) -> (19.8, -8)
  line L17 (19.8, -8) -> (14, -11.25)
  line L18 (14, -11.25) -> (12, -11.25)
  line L19 (12, -11.25) -> (12, -6.75)
  line L20 (12, -6.75) -> (16.8, -6.75)
  line L21 (16.8, -6.75) -> (16.8, -5.25)
  line L22 (12, -0.75) -> (12, 0)
  line L23 (12, -11.25) -> (12, -12)
  constraint coincident L1.end L2.start
  constraint coincident L5 L22.end
  constraint perpendicular L5 L22
  constraint coincident L18.end L19.start
  constraint coincident L15 L23.end
  constraint perpendicular L15 L23
move_body "Verschieben11" bodies 4 to x (1, 0, 0) y (0, 1, 0) z (0, 0, 1) at (53, 0, 0)
sketch "Skizze14" plane through (0, 0, 0) normal (0, -1, 0) x (1, 0, 0)
  arc A0 (-52, -8.25) -> (-52, -3.75) centre (-52, -6) ccw
  line L0 (-52, -8.25) -> (-53, -8.25)
  line L1 (-53, -8.25) -> (-53, -12)
  line L2 (-53, -12) -> (-52, -12)
  line L3 (-52, -12) -> (-52, -13)
  line L4 (-52, -13) -> (-46, -13)
  line L5 (-46, -13) -> (-46, 1)
  line L6 (-46, 1) -> (-52, 1)
  line L7 (-52, 1) -> (-52, 0)
  line L8 (-52, 0) -> (-53, 0)
  line L9 (-53, 0) -> (-53, -3.75)
  line L10 (-53, -3.75) -> (-52, -3.75)
  circle A1 centre (-52, -6) radius 2.6899
  circle A2 centre (-52, -6) radius 2.25
  line L11 (-53, -3.75) -> (-53, -8.4971)
  constraint concentric A0 A1
  constraint concentric A1 A2
  constraint coincident L9.end L10.start
  constraint coincident A1 L11.end
  constraint coincident L1 L11.end
extrude "Extrusion58" add sketch "Skizze14" against normal blind 2 contours A0 L0 L1 L9 L10 A1 A2 L11 | L0 A2 L11 | L1 L9 A1 A2 L11 | L10 A2 L11 bodies 3
extrude "Extrusion59" cut sketch "Skizze14" against normal blind 2.1 contours L1 L9 A1 A2 L11 bodies 3
move_body "Verschieben12" bodies 4 to x (1, 0, 0) y (0, 1, 0) z (0, 0, 1) at (-7, 0, 0)
extrude "Extrusion60" add 1 faces at (-60.6667, 16.8, -6.25) along direction (0, 1, 0) blind 1.5 on bodies 4 bodies 4
move_body "Verschieben13" bodies 3 to x (1, 0, 0) y (0, 1, 0) z (0, 0, 1) at (12, 0, 0)
extrude "Extrusion61" cut sketch "Skizze10" along normal blind 13 contours A6 bodies 4
extrude "Extrusion62" cut sketch "Skizze12" along normal blind 12 contours A0 bodies 4
extrude "Extrusion63" add 4 faces at (-37, 20.6473, -1.8137) (-37, 20.6436, -9.8634) (-37, 53.1467, -4.1328) (-37, 54.2878, -8.4331) along direction (1, 0, 0) blind 3 on bodies 3 bodies 3
chamfer "Fase4" distance 2 angle 45 6 edges at (-34, 53.7323, -2.3616) (-34, 23.7323, -2.3616) (-34, 23.7323, -10.3616) (-34, 7.9323, -2.3616) (-34, 7.9323, -10.3616) (-34, 53.7323, -10.3616) on bodies 3
chamfer "Fase5" distance 0.5 angle 45 18 edges at (-42, 52.8, 0) (-42, 56.4, -2) (-42, 37.8, -2) (-42, 58, -3) (-42, 22.8, 0) (-42, 20.3, -2) (-42, 19.8, -3) (-42, 58, -9) (-42, 56.4, -10) (-42, 52.8, -12) (-42, 37.8, -10) (-42, 22.8, -12) (-42, 20.3, -10) (-42, 19.8, -9) (-41, 19.2142, -0.5858) (-41, 8.9, 0) (-41, 19.2142, -11.4142) (-41, 8.9, -12) on bodies 3
chamfer "Fase6" distance 0.5 angle 45 14 edges at (-59, 22.8, 0) (-59, 20.3, -2) (-59, 19.2142, -0.5858) (-59, 8.9, 0) (-59, 37.8, -2) (-59, 52.8, 0) (-59, 56.4, -2) (-59, 56.4, -10) (-59, 52.8, -12) (-59, 37.8, -10) (-59, 22.8, -12) (-59, 20.3, -10) (-59, 19.2142, -11.4142) (-59, 8.9, -12) on bodies 4
delete_face "Fläche löschen1" 1 faces at (9.8333, 21.7355, 0.0764) on bodies 1
delete_face "Fläche löschen2" 1 faces at (9.8333, 50.94, -0.5911) on bodies 1
sketch "Skizze15" plane through (0, 0, 0) normal (1, 0, 0) x (0, 1, 0)
  line L0 (0, 0) -> (-12, 0) construction
  line L1 (-12, 12) -> (-12, 50)
  line L2 (-12, 50) -> (0, 50)
  line L3 (0, 50) -> (0, 0)
  line L4 (0, 0) -> (38, 0)
  line L5 (38, 0) -> (38, 12)
  line L6 (38, 12) -> (-12, 12)
  line L7 (-12, 12) -> (-12, 0) construction
  line L8 (-12, 0) -> (4.9706, 0) construction
  line L9 (-6, 6) -> (-12, 12) construction
  line L10 (-6, 6) -> (-16.6066, -4.6066) construction
  line L11 (-16.6066, -4.6066) -> (-10.6066, -10.6066)
  line L12 (-16.6066, -4.6066) -> (-22.6066, 1.3934)
  line L13 (0, 0) -> (-6, 6) construction
  line L14 (-12, 12) -> (-22.6066, 1.3934)
  line L15 (0, 0) -> (-10.6066, -10.6066)
  line L16 (-22.6066, 1.3934) -> (-21.8995, 2.1005)
  line L17 (-21.8995, 2.1005) -> (-9.8995, -9.8995)
  line L18 (-21.8995, 2.1005) -> (-20.4146, 3.5854)
  line L19 (-20.4146, 3.5854) -> (-8.4146, -8.4146)
  line L20 (-20.4146, 3.5854) -> (-15.1113, 8.8887)
  line L21 (-15.1113, 8.8887) -> (-3.1113, -3.1113)
  dimension "d219" = 1
  dimension "d220" = 2.1
  dimension "d221" = 7.5
  constraint horizontal L0
  constraint vertical L1
  constraint horizontal L2
  constraint vertical L3
  constraint coincident L0.start L3.end
  constraint horizontal L4
  constraint vertical L5
  constraint horizontal L6
  constraint vertical L7
  constraint horizontal L8
  constraint coincident L3 L0.start
  constraint perpendicular L12 L14
  constraint perpendicular L11 L15
  constraint perpendicular L12 L16
  constraint coincident L15 L17.end
  constraint perpendicular L15 L17
  constraint perpendicular L17 L18
  constraint coincident L15 L19.end
  constraint perpendicular L15 L19
  constraint perpendicular L19 L20
  constraint coincident L15 L21.end
  constraint perpendicular L15 L21
  measures "d219" distance of L12.end L16.end
  measures "d220" distance of L16.end L18.end
  measures "d221" distance of L18.end L20.end
extrude "Extrusion64" add sketch "Skizze15" along normal blind 6 separate body makes body 5
sketch "Skizze16" plane through (0, -10.6066, -10.6066) normal (0, -0.707107, -0.707107) x (1, 0, 0)
  line L0 (0, 16.9706) -> (0, 0)
  line L1 (0, 0) -> (6, 0)
  line L2 (6, 0) -> (6, 16.9706)
  line L3 (6, 16.9706) -> (0, 16.9706)
  line L4 (6, 16.9706) -> (5, 16.9706)
  line L5 (6, 8.4853) -> (0, 8.4853)
  line L6 (5, 8.4853) -> (5, 11.3485)
  line L7 (0, 8.4853) -> (0, 14.2353)
  line L8 (0, 8.4853) -> (0, 2.7353)
  line L9 (0, 2.7353) -> (9.0117, 2.7353) construction
  line L10 (0, 14.2353) -> (9.3871, 14.2353) construction
  line L11 (0, 14.2353) -> (5, 11.3485)
  line L12 (0, 2.7353) -> (5, 5.622)
  line L13 (5, 16.9706) -> (5, 11.3485)
  line L14 (5, 5.622) -> (5, 0)
  line L15 (5, 8.4853) -> (5, 5.622)
  line L16 (5, 11.3485) -> (5, 8.4853)
  line L17 (5, 11.3485) -> (5, 14.2353)
  line L18 (0, 14.2353) -> (-5, 11.3485)
  line L19 (-5, 11.3485) -> (-5, 8.4853)
  line L20 (-5, 8.4853) -> (-5, 5.622)
  line L21 (0, 2.7353) -> (-5, 5.622)
  circle A0 centre (0, 8.4853) radius 3.5
  circle A1 centre (0, 8.4853) radius 4
  line L22 (3.5, 8.4853) -> (3.5, 10.4218)
  line L23 (3.5, 8.4853) -> (3.5, 6.5488)
  line L24 (-3.5, 8.4853) -> (-3.5, 10.4218)
  line L25 (-3.5, 8.4853) -> (-3.5, 6.5488)
  circle A2 centre (0, 8.4853) radius 3
  point P0 (0, 8.4853)
  dimension "d224" = 1
  dimension "d225" = 5.75
  dimension "d226" = 5.75
  dimension "d227" = 5.75
  dimension "d233" = 7
  dimension "d238" = 8
  dimension "d245" = 6
  constraint coincident L2.end L3.start
  constraint perpendicular L2 L4
  constraint midpoint L2 L5.start
  constraint coincident P0 L5.end
  constraint coincident L5 L6.start
  constraint perpendicular L5 L6
  constraint perpendicular L5 L7
  constraint perpendicular L5 L8
  constraint horizontal L9
  constraint horizontal L10
  constraint coincident L1 L14.end
  constraint perpendicular L1 L13
  constraint coincident L12.end L13
  constraint perpendicular L5 L17
  constraint symmetric L6.start L7 L19.end
  constraint symmetric L10.start L7 L11.start
  constraint symmetric L7 L8.end L9.start
  constraint symmetric L7 L6.end L18.end
  constraint symmetric L7 L12.end L20.end
  constraint concentric A0 A1
  constraint coincident A0 L22.start
  constraint coincident L5 L22.start
  constraint coincident A1 L22.end
  constraint tangent A0 L22
  constraint coincident A1 L23.end
  constraint tangent A0 L23
  constraint coincident A0 L24.start
  constraint tangent A0 L24
  constraint parallel L8 L24
  constraint coincident A1 L25.end
  constraint tangent A0 L25
  constraint concentric A1 A2
  measures "d224" distance of L2.end L4.end
  measures "d225" distance of L6.start L17.end
  measures "d226" distance of P0 L7.end
  measures "d227" distance of P0 L8.end
  measures "d233" diameter of A0
  measures "d238" diameter of A1
  measures "d245" diameter of A2
extrude "Extrusion65" cut sketch "Skizze16" against normal blind 2.5 from surface at -1 contours L0 L5 L6 L7 L11 L16 A1 | L0 L7 A0 A1 L22 | L0 L5 L7 A0 A2 | L5 A1 L22 | L0 L5 L8 L12 L15 A1 | L0 L5 L7 A2 | L0 L5 L8 A0 A2 | L0 L8 A0 A1 L23 | L5 A1 L23 | L0 L5 L8 A2 bodies 5
extrude "Extrusion67" cut sketch "Skizze16" against normal blind 1 contours L0 L5 L7 A0 A2 | L0 L5 L7 A2 | L0 L5 L8 A0 A2 | L0 L5 L8 A2 bodies 5
extrude "Extrusion69" cut sketch "Skizze16" against normal blind 8 from surface at -3.5 contours L0 L7 A0 A1 L22 | L0 L5 L7 A0 A2 | L0 L5 L7 A2 | L0 L5 L8 A0 A2 | L0 L8 A0 A1 L23 | L0 L5 L8 A2 bodies 5
extrude "Extrusion71" cut sketch "Skizze16" against normal blind 2 from surface at -11.5 contours L0 L5 L7 A2 | L0 L5 L8 A2 bodies 5